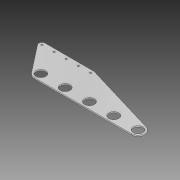
# Autodesk Inventor part: GreyT Claw 2 Wing Plate
Saved by Autodesk Inventor 2023 (Build 270158000, 158)
## iProperties
Created: 2022-01-08
Part Number: GreyT Claw 2 Wing Plate
Material: Generic
Document SubType Name: Modeling
Density: 1 g/cm^3
Appearance: Default
Appearance: Aluminum - Dark
Mass: 79.1764 g
Surface Area: 540.771 cm^2
Volume: 79.1764 cm^3
Mass: 203.115 g
Surface Area: 520.605 cm^2
Volume: 75.2277 cm^3
Density: 2.7 g/cm^3
Autodesk Inventor part; units mm, degrees
ref_plane "YZ Plane" through (0, 0, 0) normal (1, 0, 0) x (0, 1, 0)
ref_plane "XZ Plane" through (0, 0, 0) normal (0, 1, 0) x (-1, 0, 0)
ref_plane "XY Plane" through (0, 0, 0) normal (0, 0, 1) x (1, 0, 0)
sketch "Sketch1" plane through (0, 0, 0) normal (0, 1, 0) x (-1, 0, 0)
  circle A0 centre (0, 0) radius 14.2875
  line L0 (0, 0) -> (-9.1805, 0) construction
  circle A1 centre (-69.85, 0) radius 14.2875
  circle A2 centre (-139.7, 0) radius 14.2875
  circle A3 centre (-209.55, 0) radius 14.2875
  line L1 (-69.85, 0) -> (0, 0) construction
  line L2 (-69.85, -16.1701) -> (0, -16.1701) construction
  line L3 (0, 16.1701) -> (-69.85, 16.1701) construction
  arc A4 (-69.85, 16.1701) -> (-69.85, -16.1701) centre (-69.85, 0) ccw construction
  arc A5 (0, -16.1701) -> (0, 16.1701) centre (0, 0) ccw construction
  circle A6 centre (-279.4, 0) radius 14.2875
  arc A7 (15.0264, 11.7094) -> (0, 19.05) centre (0, 0) ccw
  line L4 (0, 19.05) -> (-279.4, 19.05)
  arc A8 (-279.4, 19.05) -> (-284.8345, -18.2584) centre (-279.4, 0) ccw
  line L5 (-284.8345, -18.2584) -> (-72.3716, -81.4969)
  circle A9 centre (69.85, -73.025) radius 2.4892
  line L6 (69.85, -73.025) -> (7.0465, -73.025) construction
  circle A10 centre (34.925, -73.025) radius 2.4892
  circle A11 centre (0, -73.025) radius 2.4892
  circle A12 centre (-34.925, -73.025) radius 2.4892
  circle A13 centre (-69.85, -73.025) radius 2.4892
  arc A14 (-72.3716, -81.4969) -> (-69.85, -81.8642) centre (-69.85, -73.025) ccw
  line L7 (-69.85, -81.8642) -> (69.85, -81.8642)
  arc A15 (69.85, -81.8642) -> (76.8222, -67.5918) centre (69.85, -73.025) ccw
  line L8 (76.8222, -67.5918) -> (15.0264, 11.7094)
  point P0 (-34.925, 0)
  dimension "d0" = 28.575
  dimension "d3" = 69.85
  dimension "d8" = 32.3403
  dimension "d9" = 50.8
  dimension "d10" = 69.85
  dimension "d11" = 50.8
  dimension "d12" = 69.85
  dimension "d13" = 4.7625
  dimension "d14" = 279.4
  dimension "d15" = 4.9784
  dimension "d18" = 34.925
  dimension "d23" = 6.35
  dimension "d24" = 73.025
  constraints: 20 end point, 16 centre point, 12 point on circle, 10 tangent, 7 horizontal, 2 coincident, 2 equal radius, 1 horizontal alignment, 1 midpoint, 1 parallel, 1 vertical alignment, 16 other
  measures "d0" diameter of A0
  measures "d3" distance of L0.start L1.start
  measures "d8" diameter of A5
  measures "d10" distance of L3.start L3.end
  measures "d12" distance of L2.start L2.end
  measures "d13" radial gap between concentric circles of A0 A7
  measures "d14" distance of A8.centre point (0, 0)
  measures "d15" diameter of A9
  measures "d18" distance of L6.start A10.centre
  measures "d23" radial gap between concentric circles of A13 A14
  measures "d24" distance of A11.centre point (0, 0)
extrude "Extrusion1" add sketch "Sketch1" along normal blind 3.175
extrude "Extrusion2" [suppressed]
body "Solid1"
